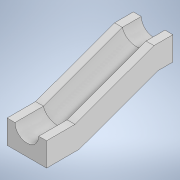
# Autodesk Inventor part: ramp(1)
Saved by Autodesk Inventor 2021 (Build 250183000, 183)
## iProperties
Created: 2021-03-26
Part Number: ramp(1)
Material: Generic
Document SubType Name: Modeling
Designer: jtri402
Density: 1 g/cm^3
Appearance: Default
Author: jtri402
Autodesk Inventor part; units mm, degrees
ref_plane "YZ Plane" through (0, 0, 0) normal (1, 0, 0) x (0, 1, 0)
ref_plane "XZ Plane" through (0, 0, 0) normal (0, 1, 0) x (-1, 0, 0)
ref_plane "XY Plane" through (0, 0, 0) normal (0, 0, 1) x (1, 0, 0)
sketch "Sketch1" plane through (0, 0, 0) normal (1, 0, 0) x (0, 1, 0)
  line L0 (0, 0) -> (0, 10)
  line L1 (0, 10) -> (-18.1985, 60)
  line L2 (-18.1985, 60) -> (-18.1985, 80)
  point P0 (0, 0)
  dimension "d6" = 0
  dimension "d7" = 0
  dimension "d8" = 10
  dimension "d15" = 20
  dimension "d16" = 50
  dimension "d17" = 20
  constraints: 6 end point, 2 vertical
  measures "d6" distance of point (0, 0) L0.start
  measures "d7" distance of point (0, 0) L0.start
  measures "d8" distance of L0.start L0.end
  measures "d15" angle of L0 L1
  measures "d16" vertical distance of L0.end L1.end
  measures "d17" distance of L1.end L2.end
sketch "Sketch2" plane through (0, 0, 0) normal (0, 0, 1) x (1, 0, 0)
  arc A0 (-7.5, 11.25) -> (7.5, 11.25) centre (0, 11.25) ccw
  line L0 (-7.5, 11.25) -> (-12.5, 11.25)
  line L1 (-12.5, 11.25) -> (-12.5, -3.75)
  line L2 (-12.5, -3.75) -> (12.5, -3.75)
  line L3 (7.5, 11.25) -> (12.5, 11.25)
  line L4 (12.5, 11.25) -> (12.5, -3.75)
  point P0 (0, 0)
  dimension "d0" = 7.5
  dimension "d20" = 15
  dimension "d21" = 5
  dimension "d22" = 5
  dimension "d23" = 25
  dimension "d30" = 3.75
  dimension "d31" = 11.25
  constraints: 10 end point, 2 horizontal, 2 perpendicular, 2 point on circle, 1 centre point
  measures "d0" radius of A0
  measures "d20" distance of L3.start L0.start
  measures "d21" distance of L3.start L3.end
  measures "d22" distance of L0.start L0.end
  measures "d23" distance of L1.end L2.end
  measures "d30" distance from line of L2 point (0, 0)
  measures "d31" distance of A0.centre point (0, 0)
sweep "Sweep3" add profiles "Sketch2" path "Sketch1"
body "Solid3"
